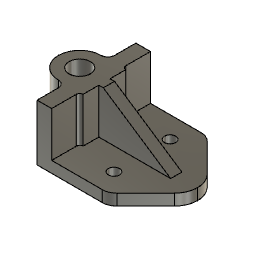
A3 v2 (Autodesk Fusion 360 design; units mm, degrees)
Autodesk Fusion 360 part; units mm, degrees
sketch "bottom" plane through (0, 0, 0) normal (0, 0, 1) x (1, 0, 0)
  line L0 (49.5, 44) -> (-49.5, 44)
  line L1 (-49.5, 44) -> (-49.5, -44)
  line L2 (-49.5, -44) -> (49.5, -44)
  line L3 (49.5, -44) -> (49.5, 44)
  line L4 (49.5, 44) -> (-49.5, -44) construction
  line L5 (-49.5, 44) -> (49.5, -44) construction
  dimension "d1" = 99
  dimension "d2" = 88
  constraint horizontal L0
  constraint perpendicular L0 L1
  constraint parallel L0 L2
  constraint parallel L1 L3
  constraint coincident L4 origin
  constraint coincident L5 origin
  measures "d1" distance of L0.start L0.end
  measures "d2" distance of L0.end L1.end
extrude "Extrude1" add sketch "bottom" along normal blind 10
sketch "circle_top" plane through (0, 0, 10) normal (0, 0, 1) x (-1, 0, 0)
  line L0 (-49.5, 44) -> (-49.5, -44)
  line L1 (-49.5, -44) -> (49.5, -44)
  line L2 (49.5, -44) -> (49.5, 44)
  line L3 (49.5, 44) -> (-49.5, 44)
  line L4 (-49.5, 0) -> (-30.5, 0) construction
  circle A0 centre (-30.5, 0) radius 19 construction
  dimension "d5" = 38
  constraint midpoint L0 L4.start
  constraint perpendicular L0 L4
  constraint coincident L4.end A0.centre
  measures "d5" diameter of A0
chamfer "Chamfer1" distance 35.5 angle 45 2 edges at (49.5, -44, 5) (49.5, 44, 5)
fillet "Fillet1" radius 20.5 2 edges at (49.5, 8.5, 5) (49.5, -8.5, 5)
fillet "Fillet2" radius 13 1 edges at (14, -44, 5)
fillet "Fillet3" radius 13 1 edges at (14, 44, 5)
sketch "wall" plane through (0, 0, 10) normal (0, 0, 1) x (-1, 0, 0)
  line L0 (49.5, 44) -> (36.5, 44)
  line L1 (36.5, 44) -> (36.5, -44)
  line L2 (36.5, -44) -> (49.5, -44)
  line L3 (49.5, -44) -> (49.5, 44)
  dimension "d13" = 13
  constraint horizontal L0
  constraint vertical L1
  constraint horizontal L2
  constraint vertical L3
  measures "d13" distance of L1.end L2.end
extrude "Extrude2" add sketch "wall" along normal blind 40
sketch "midd_wall" plane through (-36.5, 0, 0) normal (1, 0, 0) x (0, 1, 0)
  line L0 (-44, 10) -> (44, 10)
  line L1 (44, 10) -> (44, 50)
  line L2 (44, 50) -> (-44, 50)
  line L3 (-44, 50) -> (-44, 10)
  line L4 (-19, 50) -> (-19, 10)
  line L5 (19, 50) -> (19, 10)
  dimension "d16" = 38
  dimension "d17" = 25
  constraint coincident L2 L4.start
  constraint coincident L0 L4.end
  constraint perpendicular L0 L4
  constraint coincident L2 L5.start
  constraint coincident L0 L5.end
  constraint perpendicular L0 L5
  measures "d16" distance of L4 L5
  measures "d17" distance of L1 L5
extrude "Extrude3" add sketch "midd_wall" along normal blind 3 contours L0 L2 L4 L5
fillet "Fillet4" radius 3 1 edges at (-36.5, -19, 30)
fillet "Fillet5" radius 3 1 edges at (-36.5, 19, 30)
sketch "Sketch5" plane through (-33.5, 0, 0) normal (1, 0, 0) x (0, 1, 0)
  line L0 (-19, 50) -> (-19, 10)
  line L1 (-19, 10) -> (19, 10)
  line L2 (19, 10) -> (19, 50)
  line L3 (19, 50) -> (-19, 50)
  line L4 (-5, 50) -> (-5, 10)
  line L5 (5, 50) -> (5, 10)
  dimension "d24" = 10
  dimension "d25" = 14
  constraint coincident L3 L4.start
  constraint coincident L1 L4.end
  constraint perpendicular L1 L4
  constraint coincident L3 L5.start
  constraint coincident L1 L5.end
  constraint perpendicular L1 L5
  measures "d24" distance of L4 L5
  measures "d25" distance of L2 L5
extrude "Extrude4" add sketch "Sketch5" along normal blind 4 contours L1 L3 L4 L5
sketch "triangle" plane through (0, 0, 0) normal (0, 1, 0) x (1, 0, 0)
  line L0 (-29.5, -10, -5) -> (30.5, -10, -5)
  line L1 (-29.5, -10, -5) -> (-29.5, -50, -5)
  line L2 (-29.5, -50, -5) -> (30.5, -10, -5)
  dimension "d28" = 60
  dimension "d29" = 40
extrude "Extrude5" add sketch "triangle" along normal blind 10 contours L0 L1 L2 in plane through (0, -5, 0) normal (0, 1, 0)
sketch "back_tube" plane through (0, 0, 0) normal (0, 0, 1) x (1, 0, 0)
  line L0 (-49.5, -44) -> (-49.5, -19)
  line L1 (-49.5, 44) -> (-49.5, 19)
  line L2 (-49.5, -19) -> (-55.5, -19)
  line L3 (-55.5, 19) -> (-49.5, 19)
  line L4 (-49.5, 19) -> (-49.5, -19)
  circle A0 centre (-55.5, 0) radius 9.5
  arc A1 (-55.5, 19) -> (-55.5, -19) centre (-55.5, 0) ccw
  dimension "d32" = 6
  dimension "d33" = 19
  dimension "d34" = 19
  constraint vertical L0
  constraint vertical L1
  constraint horizontal L2
  constraint horizontal L3
  constraint vertical L4
  constraint concentric A0 A1
  measures "d32" distance of L0.end L2.end
  measures "d33" diameter of A0
  measures "d34" radius of A1
extrude "Extrude6" add sketch "back_tube" along normal blind 40 contours L2 L3 L4 A0 A1
extrude "Extrude7" add 1 faces at (-52.725, 15.737, 40) along direction (0, 0, 1) blind 10
extrude "Extrude8" cut sketch "back_tube" along normal blind 50 contours L4 A0 picked at (-48.8713, -1.7657)
fillet "Fillet6" radius 6 2 edges at (-49.5, 19, 25) (-49.5, -19, 25)
sketch "bottom_circles" plane through (0, 0, 10) normal (0, 0, 1) x (-1, 0, 0)
  line L0 (-30.5, 5) -> (33.5, 5)
  line L1 (33.5, 5) -> (33.5, 19)
  arc A0 (33.5, 19) -> (36.5, 22) centre (33.5, 22) ccw
  line L2 (36.5, 22) -> (36.5, 44)
  line L3 (36.5, 44) -> (-8.6152, 44)
  arc A1 (-8.6152, 44) -> (-17.8076, 40.1924) centre (-8.6152, 31) ccw
  line L4 (-17.8076, 40.1924) -> (-43.4957, 14.5043)
  arc A2 (-43.4957, 14.5043) -> (-49.5, 0.0086) centre (-29, 0.0086) ccw
  line L5 (-49.5, 0.0086) -> (-49.5, -0.0086)
  arc A3 (-49.5, -0.0086) -> (-43.4957, -14.5043) centre (-29, -0.0086) ccw
  line L6 (-43.4957, -14.5043) -> (-17.8076, -40.1924)
  arc A4 (-17.8076, -40.1924) -> (-8.6152, -44) centre (-8.6152, -31) ccw
  line L7 (-8.6152, -44) -> (36.5, -44)
  line L8 (36.5, -44) -> (36.5, -22)
  arc A5 (36.5, -22) -> (33.5, -19) centre (33.5, -22) ccw
  line L9 (33.5, -19) -> (33.5, -5)
  line L10 (33.5, -5) -> (-30.5, -5)
  line L11 (-30.5, -5) -> (-30.5, 5)
  circle A6 centre (0, 25) radius 5
  circle A7 centre (0, -25) radius 5
  dimension "d43" = 10
  dimension "d44" = 10
  measures "d43" diameter of A6
  measures "d44" diameter of A7
extrude "Extrude9" cut sketch "bottom_circles" against normal blind 10 contours A6 | A7
